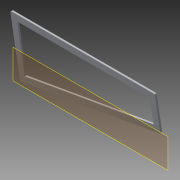
# Autodesk Inventor part: Panel_side
Saved by Autodesk Inventor 2013 (Build 170138000, 138)
## iProperties
Created: 2013-01-31
Part Number: Panel_side
Material: Aluminum 6061
Document SubType Name: Modeling
Designer: xylzlyx
Density: 1 g/cm^3
Author: xylzlyx
Autodesk Inventor part; units mm, degrees
ref_plane "YZ Plane" through (0, 0, 0) normal (1, 0, 0) x (0, 1, 0)
ref_plane "XZ Plane" through (0, 0, 0) normal (0, 1, 0) x (-1, 0, 0)
ref_plane "XY Plane" through (0, 0, 0) normal (0, 0, 1) x (1, 0, 0)
ref_plane "OriginPanel" through (0, 0, 0) normal (0, 0, 1) x (1, 0, 0)
sketch "Sketch1" plane through (0, 0, 0) normal (0, 0, 1) x (1, 0, 0)
  line L0 (-11.9302, 53.3168) -> (-257.9302, 53.3168) projected
  line L1 (-1.9696, -0.3473) -> (-241.005, -42.4957) projected
  line L2 (-257.9302, 53.3168) -> (-241.005, -42.4957)
  line L3 (-1.9696, -0.3473) -> (-11.9302, 53.3168)
  line L4 (-11.9302, 53.3168) -> (-257.9302, 53.3168)
  line L5 (-241.005, -42.4957) -> (-1.9696, -0.3473)
  point P0 (0, 0)
  constraints: 8 end point, 1 collinear
extrude "PanelExtrusion" add sketch "Sketch1" against normal blind 3
fillet "CornerFillet" radius 2 4 edges at (-257.9302, 53.3168, -1.5) (-11.9302, 53.3168, -1.5) (-1.9696, -0.3473, -1.5) (-241.005, -42.4957, -1.5)
sketch "Sketch2" plane through (0, 0, 0) normal (0, 0, 1) x (1, 0, 0)
  line L0 (-239.036, -42.1485) -> (-3.957, -0.6977) projected
  line L1 (-2.3379, 1.6369) -> (-11.6267, 51.6818) projected
  line L2 (-13.5931, 53.3168) -> (-255.5459, 53.3168) projected
  line L3 (-257.5154, 50.9689) -> (-241.3528, -40.5268) projected
  line L4 (-246.0089, 43.3168) -> (-232.8965, -30.9117)
  line L5 (-232.8965, -30.9117) -> (-13.6431, 7.7486)
  line L6 (-13.6431, 7.7486) -> (-20.2449, 43.3168)
  line L7 (-20.2449, 43.3168) -> (-246.0089, 43.3168)
  point P0 (0, 0)
  dimension "d3" = 10
  dimension "d4" = 10
  dimension "d5" = 10
  dimension "d6" = 10
  dimension "d7" = 10
  dimension "d8" = 10
  dimension "d9" = 10
  dimension "d10" = 10
  constraints: 8 end point
  measures "d3" distance from line of L3 L4.start
  measures "d4" distance from line of L3 L4.end
  measures "d5" distance from line of L2 L4.start
  measures "d6" distance from line of L2 L6.end
  measures "d7" distance from line of L1 L6.end
  measures "d8" distance from line of L1 L5.end
  measures "d9" distance from line of L0 L5.end
  measures "d10" distance from line of L0 L4.end
extrude "Extrusion2" cut sketch "Sketch2" against normal blind 3
sketch "Sketch3" plane through (0, 0, 0) normal (0, 0, 1) x (1, 0, 0)
  line L0 (-13.6431, 7.7486) -> (-232.8965, -30.9117) projected
  line L1 (-232.8965, -30.9117) -> (-246.0089, 43.3168) projected
  line L2 (-246.0089, 43.3168) -> (-20.2449, 43.3168) projected
  line L3 (-20.2449, 43.3168) -> (-13.6431, 7.7486) projected
  line L4 (-232.8965, -30.9117) -> (-20.2449, 43.3168) construction
  line L5 (-13.6431, 7.7486) -> (-246.0089, 43.3168) construction
  line L6 (-233.6014, -26.921) -> (-32.3822, 43.3168)
  line L7 (-208.3693, -26.5869) -> (-19.5064, 39.3379)
  line L8 (-245.2742, 39.1578) -> (-25.9279, 5.5825)
  line L9 (-14.4161, 11.9135) -> (-219.5727, 43.3168)
  point P0 (0, 0)
  dimension "d13" = 4
  dimension "d14" = 4
  dimension "d15" = 4
  dimension "d16" = 4
  constraints: 12 end point, 8 point on line, 4 parallel
  measures "d13" distance between parallel lines of L6 L4
  measures "d14" distance between parallel lines of L4 L7
  measures "d15" distance between parallel lines of L5 L9
  measures "d16" distance between parallel lines of L5 L8
extrude "Extrusion3" add sketch "Sketch3" against normal blind 3 contours L0 L8 L7 L9 L3 | L0 L1 L6 L8 L7 | L8 L6 L9 L7 | L7 L9 L6 L2 L3 | L8 L1 L2 L9 L6
fillet "Fillet2" radius 2 12 edges at (-233.6014, -26.921, -1.5) (-245.2742, 39.1578, -1.5) (-105.5631, 17.7722, -1.5) (-88.6883, 15.1892, -1.5) (-89.4454, 23.3983, -1.5) (-72.5706, 20.8152, -1.5) (-25.9279, 5.5825, -1.5) (-14.4161, 11.9135, -1.5) (-19.5064, 39.3379, -1.5) (-32.3822, 43.3168, -1.5) (-219.5727, 43.3168, -1.5) (-208.3693, -26.5869, -1.5)
body "Solid1"
